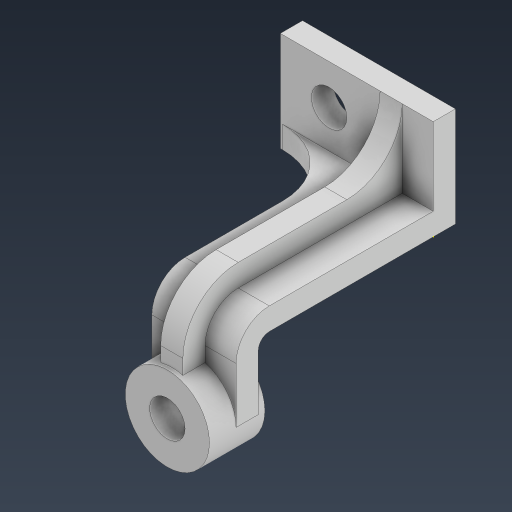
# Autodesk Inventor part: Peça teste 2
Saved by Autodesk Inventor 2024 (Build 280153000, 153)
## iProperties
Created: 2024-02-10
Part Number: Peça teste 2
Material: Genérico
Document SubType Name: Modeling
Designer: Administrator
Density: 1 g/cm^3
Appearance: Padrão
Author: Administrator
Autodesk Inventor part; units mm, degrees
ref_plane "YZ Plane" through (0, 0, 0) normal (1, 0, 0) x (0, 1, 0)
ref_plane "XZ Plane" through (0, 0, 0) normal (0, 1, 0) x (-1, 0, 0)
sketch "Esboço1" plane through (0, 0, 0) normal (1, 0, 0) x (0, 1, 0)
  line L0 (0, 0) -> (45, 0)
  line L1 (45, 0) -> (45, -10)
  line L2 (45, -10) -> (0, -10)
  line L3 (0, -10) -> (0, 0)
  dimension "d0" = 45
  dimension "d1" = 10
  constraints: 8 end point, 2 parallel, 1 horizontal, 1 perpendicular
  measures "d0" distance of L1.end L2.end
  measures "d1" distance of L0.end L1.end
extrude "Extrusão1" add sketch "Esboço1" along normal blind 69
ref_plane "Plano de trabalho1" through (0, 0, 101) normal (0, 0, 1) x (1, 0, 0)
sketch "Esboço2" plane through (0, 0, 101) normal (0, 0, 1) x (1, 0, 0)
  circle A0 centre (50, -30) radius 19
  line L0 (69, 45) -> (69, 0) projected
  line L1 (0, 45) -> (69, 45) projected
  point P0 (0, 0)
  dimension "d5" = 38
  dimension "d6" = 75
  constraints: 1 centre point, 1 tangent
  measures "d5" diameter of A0
  measures "d6" distance from line of A0.centre L1
sketch "Esboço3" plane through (69, 0, 0) normal (1, 0, 0) x (0, 0, -1)
  point P0 (0, 0)
extrude "Extrusão2" add sketch "Esboço2" against normal blind 25
sketch "Esboço4" plane through (69, 0, 0) normal (1, 0, 0) x (0, 0, -1)
  point P0 (0, 0)
sketch "Esboço5" plane through (69, 0, 0) normal (1, 0, 0) x (0, 0, -1)
  line L0 (0, 0) -> (-74, 0)
  line L1 (-79, -5) -> (-79, -30)
  line L2 (-79, -30) -> (-89, -30)
  line L3 (-89, -30) -> (-89, -5)
  line L4 (-74, 10) -> (0, 10)
  line L5 (0, 10) -> (0, 0)
  line L6 (-101, -11) -> (-101, -49) construction
  line L7 (-101, -30) -> (-76, -30) construction
  line L8 (-76, -49) -> (-76, -11) construction
  arc A0 (-74, 0) -> (-79, -5) centre (-74, -5) ccw
  arc A1 (-74, 10) -> (-89, -5) centre (-74, -5) ccw
  dimension "d9" = 10
  dimension "d10" = 3
  dimension "d11" = 5
  dimension "d12" = 15
  dimension "d20" = 12
  constraints: 14 end point, 5 perpendicular, 4 point on circle, 4 tangent, 2 centre point, 2 midpoint, 1 horizontal, 1 point on line
  measures "d9" distance between parallel lines of L0 L4
  measures "d10" distance between parallel lines of L8 L1
  measures "d11" radius of A0
  measures "d12" radius of A1
  measures "d20" distance between parallel lines of L6 L3
extrude "Extrusão3" add sketch "Esboço5" against normal blind 38
sketch "Esboço6" plane through (0, 0, 0) normal (0, 0, 1) x (1, 0, 0)
  line L0 (31, 10) -> (69, 10) projected
  line L1 (45, 10) -> (55, 10)
  line L2 (55, 10) -> (55, 20)
  line L3 (55, 20) -> (45, 20)
  line L4 (45, 20) -> (45, 10)
  line L5 (31, 10) -> (31, -5) projected
  point P0 (0, 0)
  dimension "d15" = 10
  dimension "d16" = 10
  dimension "d17" = 14
  constraints: 8 end point, 2 parallel, 1 horizontal, 1 perpendicular, 1 point on line
  measures "d15" distance of L3.end L2.end
  measures "d16" distance of L2.end L1.end
  measures "d17" distance between parallel lines of L4 L5
sketch3d "Esboço 3D1"
  line L0 (69, 10, 0) -> (69, 10, 74)
  arc A0 (69, 10, 74) -> (69, -5, 89) centre (69, -5, 74) ccw
  line L1 (69, -5, 89) -> (69, -30, 89)
sweep "Varredura1" add profiles "Esboço6" path "Esboço 3D1"
sketch "Esboço7" plane through (45, 10, 0) normal (-1, 0, 0) x (0, 0, 1)
  point P0 (0, -10)
sketch "Esboço8" plane through (45, 10, 0) normal (-1, 0, 0) x (0, 0, 1)
  point P0 (0, -10)
fillet "Arredondamento1" radius 25 1 edges at (50, 20, 0)
fillet "Arredondamento2" radius 30 1 edges at (31, 5, 0)
sketch "Esboço9" plane through (50, -30, 101) normal (0, 0, 1) x (1, 0, 0)
  circle A0 centre (0, 0) radius 19 projected
  point P0 (-50, 30)
  constraints: 1 coincident
hole "Furo1" at (50, -30, 101) direction (0, 0, -1) diameter 16 end through all
sketch "Esboço10" plane through (0, 0, 0) normal (0, 0, 1) x (1, 0, 0)
  line L0 (0, 45) -> (45, 45) projected
  line L1 (0, 45) -> (0, 0) projected
  point P0 (22, 27)
  dimension "d30" = 18
  dimension "d31" = 22
  measures "d30" distance from line of L0 point (22, 27)
  measures "d31" distance from line of L1 point (22, 27)
hole "Furo2" at (22, 27, 0) direction (0, 0, -1) diameter 16 end through all
